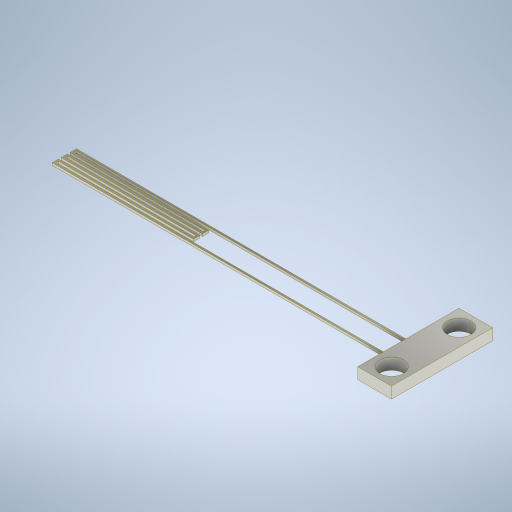
# Autodesk Inventor part: strain guage abs 9_17_2024
Saved by Autodesk Inventor 2024.2 (Build 282272000, 272)
## iProperties
Created: 2024-07-17
Part Number: strain guage abs 9_17_2024
Material: Silver
Document SubType Name: Modeling
Designer: Makerspace
Density: 10.49 g/cm^3
Appearance: Silver
Author: Makerspace
Autodesk Inventor part; units mm, degrees
ref_plane "XZ Plane" through (0, 0, 0) normal (0, 1, 0) x (-1, 0, 0)
sketch "Sketch1" plane through (0, 0, 0) normal (0, 1, 0) x (-1, 0, 0)
  line L0 (0, 0) -> (95.25, 0)
  line L1 (95.25, 0) -> (95.25, -1.27)
  line L2 (95.25, -1.27) -> (57.15, -1.27)
  line L3 (57.15, -1.27) -> (57.15, -2.54)
  line L4 (57.15, -2.54) -> (95.25, -2.54)
  line L5 (95.25, -2.54) -> (95.25, -3.81)
  line L6 (95.25, -3.81) -> (57.15, -3.81)
  line L7 (57.15, -3.81) -> (57.15, -5.08)
  line L8 (57.15, -5.08) -> (95.25, -5.08)
  line L9 (95.25, -5.08) -> (95.25, -6.35)
  line L10 (95.25, -6.35) -> (57.15, -6.35)
  line L11 (57.15, -6.35) -> (47.625, -6.35)
  line L12 (47.625, -6.35) -> (31.75, -6.35)
  line L13 (31.75, -6.35) -> (0, -6.35)
  dimension "d0" = 95.25
  dimension "d1" = 1.27
  dimension "d2" = 38.1
  dimension "d3" = 1.27
  dimension "d22" = 38.1
  dimension "d23" = 1.27
  constraints: 28 end point, 6 horizontal, 3 collinear, 3 perpendicular, 3 point on line, 3 vertical, 1 parallel
  measures "d0" distance of L0.start L0.end
  measures "d1" distance of L0.end L1.end
  measures "d2" distance of L1.end L2.end
  measures "d3" distance of L2.end L3.end
  measures "d22" distance of L5.end L6.end
  measures "d23" distance of L6.end L7.end
sketch "Sketch2" plane through (0, 0, 0) normal (1, 0, 0) x (0, 1, 0)
  line L0 (0.635, 0.635) -> (-0.635, -0.635) construction
  line L1 (-0.635, 0.635) -> (0.635, -0.635) construction
  line L2 (0.254, 0.254) -> (-0.381, 0.254)
  line L3 (-0.381, 0.254) -> (-0.381, -0.254)
  line L4 (-0.381, -0.254) -> (0.254, -0.254)
  line L5 (0.254, -0.254) -> (0.254, 0.254)
  line L6 (0.254, 0.254) -> (-0.381, -0.254) construction
  line L7 (-0.381, 0.254) -> (0.254, -0.254) construction
  point P0 (0, 0)
  dimension "d4" = 1.27
  dimension "d5" = 1.27
  dimension "d24" = 0.635
  constraints: 16 end point, 2 midpoint, 2 parallel, 1 horizontal, 1 perpendicular
  measures "d4" distance of L1.end L0.start
  measures "d5" distance of L0.start L1.start
  measures "d24" distance of L3.end L4.end
sweep "Sweep1" add profiles "Sketch2" path "Sketch1"
ref_plane "Work Plane1" through (6.35, 0, 0) normal (1, 0, 0) x (0, 1, 0)
ref_plane "Work Plane2" through (0, 0, -6.35) normal (0, 0, 1) x (1, 0, 0)
sketch "Sketch6" plane through (-95.504, -0.381, 0.254) normal (0, -1, 0) x (1, 0, 0)
  line L0 (95.504, 9.271) -> (105.029, 9.271)
  line L1 (105.029, 9.271) -> (105.029, -19.304)
  line L2 (105.029, -19.304) -> (95.504, -19.304)
  line L3 (95.504, -19.304) -> (95.504, 9.271)
  line L4 (63.754, -9.525) -> (63.754, -10.033) projected
  line L5 (95.504, 0) -> (95.504, -0.508) projected
  point P0 (95.504, -0.254)
  point P1 (63.754, -9.779)
  point P2 (105.029, -5.0165)
  point P3 (63.754, -9.779)
  point P4 (95.504, -0.254)
  dimension "d25" = 28.575
  dimension "d26" = 9.525
  dimension "d28" = 4.7625
  dimension "d29" = 0
  constraints: 8 end point, 4 midpoint, 2 parallel, 1 horizontal, 1 perpendicular
  measures "d25" distance of L0.end L1.end
  measures "d26" distance of L0.start L0.end
  measures "d28" vertical distance of point (63.754, -9.779) point (105.029, -5.017)
  measures "d29" distance from line of point (95.504, -0.254) L3
extrude "Extrusion4" add sketch "Sketch6" against normal blind 3.175
fillet "Fillet1" radius 3.175 1 edges at (0, 0.254, 0)
sketch "Sketch7" plane through (-95.504, 2.794, 0.254) normal (0, 1, 0) x (1, 0, 0)
  circle A0 centre (100.331, -4.5085) radius 3.302
  circle A1 centre (100.33, 14.5415) radius 3.302
  line L0 (105.029, 19.304) -> (95.504, 19.304) projected
  line L1 (105.029, -9.271) -> (105.029, 19.304) projected
  point P0 (95.504, 0.254)
  point P1 (70.9966, 19.304)
  point P2 (69.1826, 19.304)
  dimension "d33" = 6.604
  dimension "d34" = 6.604
  dimension "d35" = 19.05
  dimension "d36" = 4.7625
  dimension "d39" = 4.699
  dimension "d40" = 4.698
  constraints: 2 centre point
  measures "d33" diameter of A1
  measures "d34" diameter of A0
  measures "d35" distance of A1.centre A0.centre
  measures "d36" distance from line of L0 A1.centre
  measures "d39" distance from line of L1 A1.centre
  measures "d40" distance from line of L1 A0.centre
extrude "Extrusion5" cut sketch "Sketch7" against normal through all
fillet "Fillet2" radius 3.175 1 edges at (0, 0.254, -6.35)
body "Solid1"
